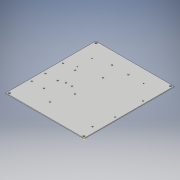
# Autodesk Inventor part: L17_TSI_008
Saved by Autodesk Inventor 2017 (Build 210142000, 142)
## iProperties
Manager: Greg Flynn
Company: Lafayette College ECE
Created: 2017-04-13
Part Number: L17_TSI_008
Material: Generic
Document SubType Name: Modeling
Designer: Christer Hoeflinger
Density: 1 g/cm^3
Appearance: Default
Project: LFEV17
Engineer: Christer Hoeflinger
Author: Christer Hoeflinger
Title: TSI Base Plate
Revision Number: 1
Autodesk Inventor part; units mm, degrees
ref_plane "YZ Plane" through (0, 0, 0) normal (1, 0, 0) x (0, 1, 0)
ref_plane "XZ Plane" through (0, 0, 0) normal (0, 1, 0) x (-1, 0, 0)
ref_plane "XY Plane" through (0, 0, 0) normal (0, 0, 1) x (1, 0, 0)
sketch "Sketch1" plane through (0, 0, 0) normal (0, 1, 0) x (-1, 0, 0)
  line L0 (0, 0) -> (327.025, 0)
  line L1 (327.025, 0) -> (327.025, -374.65)
  line L2 (327.025, -374.65) -> (0, -374.65)
  line L3 (0, -374.65) -> (0, 0)
  dimension "d0" = 374.65
  dimension "d1" = 327.025
  constraints: 8 end point, 2 parallel, 1 horizontal, 1 perpendicular
  measures "d0" distance of L0.end L1.end
  measures "d1" distance of L0.start L0.end
extrude "Extrusion1" add sketch "Sketch1" along normal blind 3.175
sketch "Sketch8" plane through (0, 3.175, 0) normal (0, 1, 0) x (1, 0, 0)
  circle A0 centre (-179.07, 140.0175) radius 1.75 projected
  circle A1 centre (-11.43, 140.0175) radius 1.75 projected
  line L0 (-184.15, 134.9375) -> (-6.35, 134.9375) projected
  line L1 (-6.35, 233.0375) -> (-184.15, 233.0375) projected
  line L2 (-184.15, 233.0375) -> (-184.15, 134.9375) projected
  line L3 (-6.35, 134.9375) -> (-6.35, 233.0375) projected
  point P0 (0, 0)
  point P1 (-179.07, 256.8575)
  point P2 (-11.43, 256.8575)
  point P3 (-11.43, 140.0175)
  point P4 (-179.07, 140.0175)
  constraints: 2 coincident
hole "Hole7" at (-179.07, 3.175, -256.8575) at (-11.43, 3.175, -256.8575) at (-11.43, 3.175, -140.0175) at (-179.07, 3.175, -140.0175) direction (0, -1, 0) diameter 5.4102 end through all
sketch "Sketch9" plane through (0, 3.175, 0) normal (0, 1, 0) x (1, 0, 0)
  circle A0 centre (-205.6765, 321.4878) radius 3.175 projected
  circle A1 centre (-137.3505, 321.4878) radius 3.175 projected
  point P0 (0, 0)
  constraints: 2 coincident
hole "Hole8" at (-205.6765, 3.175, -321.4878) at (-137.3505, 3.175, -321.4878) direction (0, -1, 0) diameter 5.4102 end through all
sketch "Sketch11" plane through (0, 3.175, 0) normal (0, 1, 0) x (1, 0, 0)
  line L0 (0, 374.65) -> (-327.025, 374.65) projected
  line L1 (0, 0) -> (0, 374.65) projected
  circle A0 centre (-205.6765, 321.4878) radius 2.7051 projected
  circle A1 centre (-137.3505, 321.4878) radius 2.7051 projected
  circle A2 centre (-11.43, 140.0175) radius 2.7051 projected
  circle A3 centre (-179.07, 256.8575) radius 2.7051 projected
  circle A4 centre (-11.43, 256.8575) radius 2.7051 projected
  circle A5 centre (-179.07, 140.0175) radius 2.7051 projected
  line L2 (-327.025, 0) -> (0, 0) projected
  line L3 (0, 0) -> (0, 374.65) projected
  line L4 (0, 374.65) -> (-327.025, 374.65) projected
  line L5 (-327.025, 374.65) -> (-327.025, 0) projected
  point P0 (-319.151, 6.35)
  point P1 (-7.874, 6.35)
  point P2 (-7.874, 368.3)
  point P3 (-319.151, 368.3)
  dimension "d85" = 6.35
  dimension "d86" = 6.35
  dimension "d87" = 7.874
  dimension "d88" = 7.874
  dimension "d89" = 6.35
  dimension "d90" = 7.874
  dimension "d91" = 7.874
  dimension "d92" = 6.35
  measures "d85" distance from line of L0 point (-319.151, 368.3)
  measures "d86" distance from line of L0 point (-7.874, 368.3)
  measures "d87" distance from line of L1 point (-7.874, 368.3)
  measures "d88" distance from line of L5 point (-319.151, 368.3)
  measures "d89" distance from line of L2 point (-7.874, 6.35)
  measures "d90" distance from line of point (-7.874, 6.35) L1
  measures "d91" distance from line of L5 point (-319.151, 6.35)
  measures "d92" distance from line of point (-319.151, 6.35) L2
hole "Hole10" at (-319.151, 3.175, -6.35) at (-7.874, 3.175, -6.35) at (-7.874, 3.175, -368.3) at (-319.151, 3.175, -368.3) direction (0, -1, 0) diameter 8.255 end through all
sketch "Sketch15" plane through (0, 3.175, 0) normal (0, 1, 0) x (1, 0, 0)
  arc A0 (-136.6, 61.3) -> (-136.6, 56.1) centre (-136.6, 58.7) ccw projected
  line L0 (-136.6, 61.3) -> (-116.8, 61.3) projected
  arc A1 (-116.8, 56.1) -> (-116.8, 61.3) centre (-116.8, 58.7) ccw projected
  line L1 (-116.8, 56.1) -> (-136.6, 56.1) projected
  arc A2 (-188.8, 56.1) -> (-188.8, 61.3) centre (-188.8, 58.7) ccw projected
  line L2 (-188.8, 56.1) -> (-208.6, 56.1) projected
  arc A3 (-208.6, 61.3) -> (-208.6, 56.1) centre (-208.6, 58.7) ccw projected
  line L3 (-208.6, 61.3) -> (-188.8, 61.3) projected
  arc A4 (-152.8, 56.1) -> (-152.8, 61.3) centre (-152.8, 58.7) ccw projected
  line L4 (-152.8, 56.1) -> (-172.6, 56.1) projected
  arc A5 (-172.6, 61.3) -> (-172.6, 56.1) centre (-172.6, 58.7) ccw projected
  line L5 (-172.6, 61.3) -> (-152.8, 61.3) projected
  line L6 (-112.7, 70.2) -> (-212.7, 70.2) projected
  line L7 (-212.7, 47.2) -> (-212.7, 70.2) projected
  line L8 (-212.7, 47.2) -> (-112.7, 47.2) projected
  line L9 (-112.7, 70.2) -> (-112.7, 47.2) projected
  arc A6 (-36.6, 61.3) -> (-36.6, 56.1) centre (-36.6, 58.7) ccw projected
  line L10 (-36.6, 61.3) -> (-16.8, 61.3) projected
  arc A7 (-16.8, 56.1) -> (-16.8, 61.3) centre (-16.8, 58.7) ccw projected
  line L11 (-16.8, 56.1) -> (-36.6, 56.1) projected
  arc A8 (-88.8, 56.1) -> (-88.8, 61.3) centre (-88.8, 58.7) ccw projected
  line L12 (-88.8, 56.1) -> (-108.6, 56.1) projected
  arc A9 (-108.6, 61.3) -> (-108.6, 56.1) centre (-108.6, 58.7) ccw projected
  line L13 (-108.6, 61.3) -> (-88.8, 61.3) projected
  arc A10 (-52.8, 56.1) -> (-52.8, 61.3) centre (-52.8, 58.7) ccw projected
  line L14 (-52.8, 56.1) -> (-72.6, 56.1) projected
  arc A11 (-72.6, 61.3) -> (-72.6, 56.1) centre (-72.6, 58.7) ccw projected
  line L15 (-72.6, 61.3) -> (-52.8, 61.3) projected
  line L16 (-12.7, 70.2) -> (-112.7, 70.2) projected
  line L17 (-112.7, 47.2) -> (-112.7, 70.2) projected
  line L18 (-112.7, 47.2) -> (-12.7, 47.2) projected
  line L19 (-12.7, 70.2) -> (-12.7, 47.2) projected
  point P0 (0, 0)
  point P1 (-202.25, 58.7)
  point P2 (-24.45, 58.7)
  dimension "d121" = 5.2
  dimension "d122" = 2.6
  dimension "d123" = 2.6
  dimension "d124" = 6.35
  dimension "d179" = 177.8
  measures "d121" distance between parallel lines of L10 L11
  measures "d122" distance from line of point (-24.45, 58.7) L11
  measures "d123" distance from line of point (-202.25, 58.7) L2
  measures "d124" distance of A3.centre point (-202.25, 58.7)
  measures "d179" distance of point (-202.25, 58.7) point (-24.45, 58.7)
hole "Hole14" at (-202.25, 3.175, -58.7) at (-24.45, 3.175, -58.7) direction (0, -1, 0) diameter 5.4102 end through all
sketch "Sketch16" plane through (0, 3.175, 0) normal (0, 1, 0) x (1, 0, 0)
  circle A0 centre (-272.2753, 243.7003) radius 1.651 projected
  circle A1 centre (-272.2753, 304.0253) radius 1.651 projected
  circle A2 centre (-272.2753, 265.9253) radius 4.7625 projected
  circle A3 centre (-272.2753, 323.0753) radius 4.7625 projected
  line L0 (-259.5753, 332.6003) -> (-259.5753, 231.0003) projected
  line L1 (-284.9753, 332.6003) -> (-259.5753, 332.6003) projected
  line L2 (-284.9753, 332.6003) -> (-284.9753, 231.0003) projected
  line L3 (-259.5753, 231.0003) -> (-284.9753, 231.0003) projected
  circle A4 centre (-73.7997, 321.4878) radius 1.651 projected
  circle A5 centre (-132.7785, 321.4878) radius 1.5 projected
  circle A6 centre (-108.7785, 321.4878) radius 1.5 projected
  line L4 (-169.291, 308.7878) -> (-169.291, 334.1878) projected
  line L5 (-169.291, 308.7878) -> (-43.6372, 308.7878) projected
  line L6 (-169.291, 334.1878) -> (-43.6372, 334.1878) projected
  line L7 (-43.6372, 334.1878) -> (-43.6372, 308.7878) projected
  circle A7 centre (-54.7497, 321.4878) radius 4.7625 projected
  circle A8 centre (-158.1785, 321.4878) radius 6.35 projected
  circle A9 centre (-86.4997, 321.4878) radius 1.651 projected
  circle A10 centre (-272.2753, 291.3253) radius 1.651 projected
  point P0 (0, 0)
  point P1 (-272.2753, 243.7003)
  constraints: 3 coincident
hole "Hole15" at (-272.2753, 3.175, -243.7003) at (-272.2753, 3.175, -304.0253) at (-73.7997, 3.175, -321.4878) direction (0, -1, 0) diameter 3.302 end through all thread size "8-32 UNC" class "2B" standard "ANSI Unified Screw Threads"
sketch "Sketch19" plane through (0, 0, 0) normal (0, -1, 0) x (1, 0, 0)
  line L0 (-19.9439, -18.4262) -> (-50.6586, -18.4262) construction
  line L1 (-50.6586, -18.4262) -> (-50.6586, -14.7014) construction
  line L2 (-50.6586, -14.7014) -> (-19.9439, -14.7014) construction
  line L3 (-19.9439, -14.7014) -> (-19.9439, -18.4262) construction
  point P0 (0, 0)
  constraints: 2 other
sketch "Sketch20" plane through (0, 3.175, 0) normal (0, 1, 0) x (1, 0, 0)
  line L0 (-327.025, 374.65) -> (-327.025, 0) projected
  line L1 (-327.025, 0) -> (0, 0) projected
  point P0 (-314.325, 95.25)
  point P1 (-263.525, 95.25)
  point P2 (-263.525, 152.4)
  point P3 (-314.325, 152.4)
  point P4 (-314.325, 225.425)
  point P5 (-263.525, 225.425)
  dimension "d147" = 50.8
  dimension "d148" = 50.8
  dimension "d149" = 50.8
  dimension "d150" = 12.7
  dimension "d151" = 12.7
  dimension "d152" = 12.7
  dimension "d153" = 95.25
  dimension "d154" = 0
  dimension "d155" = 0
  dimension "d156" = 57.15
  dimension "d157" = 130.175
  dimension "d158" = 0
  measures "d147" distance of point (-314.325, 95.25) point (-263.525, 95.25)
  measures "d148" distance of point (-314.325, 152.4) point (-263.525, 152.4)
  measures "d149" distance of point (-314.325, 225.425) point (-263.525, 225.425)
  measures "d150" distance from line of L0 point (-314.325, 95.25)
  measures "d151" distance from line of L0 point (-314.325, 152.4)
  measures "d152" distance from line of L0 point (-314.325, 225.425)
  measures "d153" distance from line of L1 point (-314.325, 95.25)
  measures "d154" vertical distance of point (-314.325, 95.25) point (-263.525, 95.25)
  measures "d155" vertical distance of point (-314.325, 152.4) point (-263.525, 152.4)
  measures "d156" distance of point (-314.325, 152.4) point (-314.325, 95.25)
  measures "d157" distance of point (-314.325, 95.25) point (-314.325, 225.425)
  measures "d158" vertical distance of point (-314.325, 225.425) point (-263.525, 225.425)
hole "Hole16" at (-314.325, 3.175, -95.25) at (-263.525, 3.175, -95.25) at (-263.525, 3.175, -152.4) at (-314.325, 3.175, -152.4) at (-314.325, 3.175, -225.425) at (-263.525, 3.175, -225.425) direction (0, -1, 0) diameter 5.4102 end through all
sketch "Sketch21" plane through (0, 3.175, 0) normal (0, 1, 0) x (1, 0, 0)
  circle A0 centre (-179.07, 256.8575) radius 2.7051 projected
  circle A1 centre (-263.525, 152.4) radius 2.7051 projected
  point P0 (0, 0)
  point P1 (-238.125, 161.6075)
  point P2 (-225.425, 161.6075)
  point P3 (-212.725, 161.6075)
  dimension "d166" = 95.25
  dimension "d167" = 0
  dimension "d168" = 0
  dimension "d169" = 38.1
  dimension "d170" = 12.7
  dimension "d171" = 12.7
  measures "d166" vertical distance of A0.centre point (-238.125, 161.608)
  measures "d167" vertical distance of point (-225.425, 161.608) point (-238.125, 161.608)
  measures "d168" vertical distance of point (-212.725, 161.608) point (-238.125, 161.608)
  measures "d169" horizontal distance of A1.centre point (-225.425, 161.608)
  measures "d170" distance of point (-225.425, 161.608) point (-238.125, 161.608)
  measures "d171" distance of point (-225.425, 161.608) point (-212.725, 161.608)
hole "Hole17" at (-238.125, 3.175, -161.6075) at (-212.725, 3.175, -161.6075) direction (0, -1, 0) diameter 5.4102 end through all
equation "\"d122\" = 0.5 * d121"
equation "\"d123\" = d122"
equation "\"d148\" = d147"
equation "\"d149\" = d147"
equation "\"d151\" = d150"
body "Solid1"
